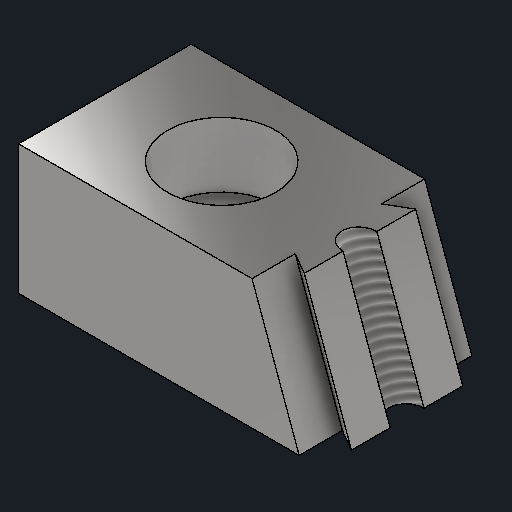
# Autodesk Inventor part: Part1
Saved by Autodesk Inventor 2026.2 (Build 302298000, 298)
## iProperties
Created: 2026-09-23
Part Number: Part1
Material: Steel, Alloy
Document SubType Name: Modeling
Designer: JoshuaEah
Density: 7.73 g/cm^3
Appearance: Semi-Polished
Author: JoshuaEah
Autodesk Inventor part; units mm, degrees
ref_plane "YZ Plane" through (0, 0, 0) normal (1, 0, 0) x (0, 1, 0)
ref_plane "XZ Plane" through (0, 0, 0) normal (0, 1, 0) x (-1, 0, 0)
sketch "Sketch1" plane through (0, 0, 0) normal (0, 1, 0) x (-1, 0, 0)
  line L0 (0, 0) -> (-44.45, 0)
  line L1 (-44.45, 0) -> (-44.45, -25.4)
  line L2 (-44.45, -25.4) -> (0, -25.4)
  line L3 (0, -25.4) -> (0, 0)
  line L4 (-41.275, -25.4) -> (-41.275, 0)
  line L5 (-41.275, -19.05) -> (-44.45, -20.8831)
  line L6 (0, -12.7) -> (-44.45, -12.7) construction
  line L7 (-41.275, -6.35) -> (-44.45, -4.5169)
  point P0 (-44.45, -4.5169)
  point P1 (-41.275, -6.35)
  dimension "d0" = 44.45
  dimension "d7" = 25.4
  dimension "d10" = 3.175
  dimension "d11" = 12.7
  dimension "d12" = 60
  constraints: 16 end point, 4 point on line, 2 midpoint, 2 parallel, 2 perpendicular, 2 symmetric about line, 1 coincident, 1 horizontal
  measures "d0" distance of L2.end L1.end
  measures "d7" distance of L2.end L0.start
  measures "d10" distance between parallel lines of L1 L4
  measures "d11" diameter of L5.start L6
  measures "d12" angle of L4 L5
extrude "Extrusion1" add sketch "Sketch1" along normal blind 19.05
sketch "Sketch3" plane through (0, 0, 0) normal (0, 0, 1) x (1, 0, 0)
  line L0 (0, 0) -> (44.45, 0) projected
  line L1 (44.45, 0) -> (44.45, 19.05) projected
  line L2 (0, 19.05) -> (44.45, 19.05) projected
  line L3 (0, 0) -> (0, 19.05) projected
  line L4 (24.8164, 19.05) -> (31.75, 0)
  dimension "d14" = 70
  dimension "d15" = 31.75
  constraints: 2 end point, 2 point on line
  measures "d14" angle of L0 L4
  measures "d15" distance from line of L3 L4.end
sweep "Sweep1" cut profiles "Sketch1" path "Sketch3" path curves L4 contours L4 L7 L1 L0 | L2 L1 L5 L4
ref_plane "Work Plane3" through (44.45, 0, 0) normal (-0.342, 0.9397, 0) x (0, 0, -1)
ref_plane "Work Plane2" through (44.45, 0, 0) normal (-0.9397, -0.342, 0) x (0, 0, -1)
sketch "Sketch5" plane through (44.45, 0, 0) normal (-0.342, 0.9397, 0) x (0, 0, -1)
  point P0 (12.7, 0)
hole "Hole2" at (44.45, 0, -12.7) direction (-0.342, 0.9397, 0) diameter 4.9784 end through all
split "Split1" plane through (44.45, 0, 0) removes the side toward (0.9397, 0.342, 0)
sketch "Sketch4" plane through (0, 19.05, 0) normal (0, 1, 0) x (1, 0, 0)
  line L0 (0, 0) -> (34.3414, 0) construction
  line L1 (0, 25.4) -> (0, 0) construction
  point P0 (17.1707, 12.7)
  point P1 (0, 12.7)
  point P2 (17.1707, 0)
  constraints: 2 midpoint, 1 horizontal alignment, 1 vertical alignment
hole "Hole1" at (17.1707, 19.05, -12.7) direction (0, -1, 0) diameter 10.0838 end through all counterbore diameter 15.875 counterbore depth 9.525
equation "\"d14\" = slopeAngle"
equation "\"d18\" = slopeAngle"
equation "\"slopeAngle\" = 70deg"
body "Solid1"
